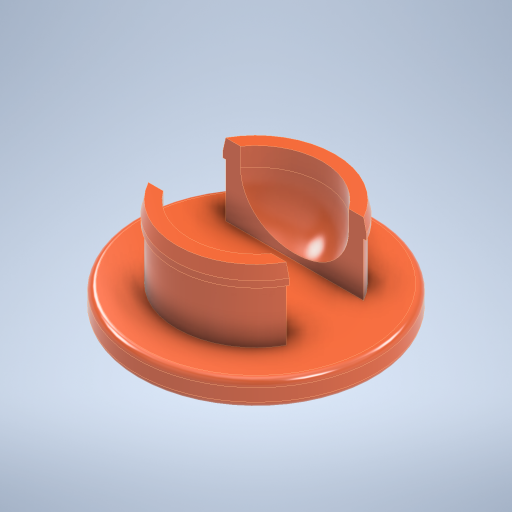
# Autodesk Inventor part: çıkçık
Saved by Autodesk Inventor 2023.2 (Build 272271000, 271)
## iProperties
Created: 2022-12-07
Part Number: çıkçık
Material: Generic
Document SubType Name: Modeling
Designer: omrfrkmll
Density: 1 g/cm^3
Appearance: Smooth - Light Orange
Author: omrfrkmll
Autodesk Inventor part; units mm, degrees
ref_plane "YZ Plane" through (0, 0, 0) normal (1, 0, 0) x (0, 1, 0)
ref_plane "XZ Plane" through (0, 0, 0) normal (0, 1, 0) x (-1, 0, 0)
ref_plane "XY Plane" through (0, 0, 0) normal (0, 0, 1) x (1, 0, 0)
sketch "Sketch1" plane through (0, 0, 0) normal (0, 0, 1) x (1, 0, 0)
  line L0 (0, 16.122948) -> (0, -13.98419)
  line L1 (0, 0) -> (9.5, 0)
  line L2 (9.5, 0) -> (9.5, 2)
  line L3 (9.5, 2) -> (6.3, 2)
  line L4 (6.3, 2) -> (6.3, 6.25)
  line L5 (6.3, 6.25) -> (6.5, 6.25)
  line L6 (6.3, 7.75) -> (0, 7.75)
  line L7 (0, 7.75) -> (0, 0)
  line L8 (0, 7.75) -> (0, 0)
  line L9 (6.5, 6.25) -> (6.5, 6.75)
  line L10 (6.5, 6.75) -> (6.3, 7.75)
  dimension "d1" = 19
  dimension "d3" = 0.2
  dimension "d5" = 5.75
  dimension "d6" = 12.6
  dimension "d12" = 1
  dimension "d13" = 0.5
  dimension "d14" = 2
  constraints: 22 end point, 4 perpendicular, 3 vertical, 2 collinear, 1 horizontal, 1 parallel, 1 point on line
  measures "d1" diameter of L2 L0
  measures "d3" distance from line of L4 L5.end
  measures "d5" distance between parallel lines of L3 L6
  measures "d6" diameter of L4 L0
  measures "d12" distance from line of L9.end L6
  measures "d13" distance from line of L5 L9.end
  measures "d14" distance between parallel lines of L1 L3
revolve "Revolution1" add sketch "Sketch1" angle 360 about axis through (0, 16.122948, 0) along (0, -1, 0)
sketch "Sketch2" plane through (0, 7.75, 0) normal (0, 1, 0) x (1, 0, 0)
  line L0 (15.51415, -3.081395) -> (15.51415, 3.081395)
  line L1 (-15.51415, 3.081395) -> (-15.51415, -3.081395)
  line L2 (-3.506868, 0) -> (2.260298, 0)
  line L3 (0, -3.176732) -> (0, 4.755286)
  circle A0 centre (0, 0) radius 6.3
  line L4 (-15.51415, -3.081395) -> (-4.312192, -3.081395)
  line L5 (4.312192, -3.081395) -> (15.51415, -3.081395)
  line L6 (15.51415, 3.081395) -> (4.312192, 3.081395)
  line L7 (-4.312192, 3.081395) -> (-15.51415, 3.081395)
  arc A1 (4.312192, -3.081395) -> (-4.312192, 3.081395) centre (0, 0) ccw
  arc A2 (-4.312192, 3.081395) -> (4.312192, -3.081395) centre (0, 0) ccw
  dimension "d15" = 5.3
  constraints: 16 end point, 6 point on circle, 5 parallel, 4 horizontal, 2 centre point, 2 perpendicular, 2 vertical, 1 coincident, 1 other
  measures "d15" radius of A1
extrude "Extrusion1" cut sketch "Sketch2" against normal up to surface (5.75 mm away) contours A2 A1
fillet "Fillet1" radius 0.5 2 edges at (-9.5, 0, 0) (-9.5, 2, 0)
fillet "Fillet2" radius 4.25 1 edges at (4.3122, 2, 3.0814)
sketch "Sketch3" plane through (0, 2, 0) normal (0, 1, 0) x (1, 0, 0)
  line L0 (-10.404923, -3.0815) -> (9.880673, -3.0815)
  line L1 (9.880673, -3.0815) -> (9.880673, 3.0815)
  line L2 (9.880673, 3.0815) -> (-10.404923, 3.0815)
  line L3 (-10.404923, 3.0815) -> (-10.404923, -3.0815)
  line L4 (-12.5563, 0) -> (12.222543, 0)
  point P0 (0, 0)
  dimension "d18" = 6.163
  constraints: 10 end point, 3 horizontal, 2 parallel, 1 perpendicular, 1 other
  measures "d18" distance between parallel lines of L2 L0
extrude "Extrusion2" cut sketch "Sketch3" along normal up to surface (5.75 mm away)
body "Solid1"
